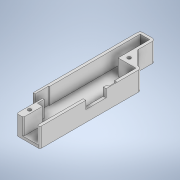
# Autodesk Inventor part: Case_DIP
Saved by Autodesk Inventor 2021 (Build 250183000, 183)
## iProperties
Created: 2021-02-15
Part Number: Case_DIP
Material: Generisch
Document SubType Name: Modeling
Designer: nostrabis
Density: 1 g/cm^3
Appearance: Vorgabe
Author: nostrabis
Autodesk Inventor part; units mm, degrees
ref_plane "YZ Plane" through (0, 0, 0) normal (1, 0, 0) x (0, 1, 0)
ref_plane "XZ Plane" through (0, 0, 0) normal (0, 1, 0) x (-1, 0, 0)
ref_plane "XY Plane" through (0, 0, 0) normal (0, 0, 1) x (1, 0, 0)
sketch "Skizze1" plane through (0, 0, 0) normal (0, 1, 0) x (-1, 0, 0)
  line L0 (0, 0) -> (10, 0)
  line L1 (20, -14) -> (20, -70)
  line L2 (13, -70) -> (0, -70)
  line L3 (0, -70) -> (0, 0)
  line L4 (20, -70) -> (13, -70)
  line L5 (13, -70) -> (13, -93)
  line L6 (13, -93) -> (20, -93)
  line L7 (20, -93) -> (20, -70)
  line L8 (20, 0) -> (10, 0)
  line L9 (10, 0) -> (10, -14)
  line L10 (10, -14) -> (20, -14)
  line L11 (20, -14) -> (20, 0)
  line L12 (20, -12) -> (12, -12)
  line L13 (12, -12) -> (12, 0)
  line L14 (10, 2) -> (-2, 2)
  line L15 (-2, 2) -> (-2, -72)
  line L16 (-2, -72) -> (13, -72)
  line L17 (11, -70) -> (11, -95)
  line L18 (11, -95) -> (22, -95)
  line L19 (22, -95) -> (22, -70)
  line L20 (10, 2) -> (12, 2)
  line L21 (12, 2) -> (12, 0)
  line L22 (20, -12) -> (22, -12)
  line L23 (22, -12) -> (22, -70)
  line L24 (10, 0) -> (10, 2)
  line L25 (0, 0) -> (0, 2)
  line L26 (10, -14) -> (20, -14)
  line L27 (20, -14) -> (20, -21)
  line L28 (20, -21) -> (10, -21)
  line L29 (10, -21) -> (10, -14)
  line L30 (12, -12) -> (12, -14)
  line L31 (20, -21) -> (22, -21)
  line L32 (20, -14) -> (22, -14)
  line L33 (12, 2) -> (15, 2)
  line L34 (15, 2) -> (15, -14)
  line L35 (15, -14) -> (12, -14)
  line L36 (12, -14) -> (12, 2)
  line L37 (10, -14) -> (15, -14)
  line L38 (15, -14) -> (15, -21)
  line L39 (15, -21) -> (10, -21)
  line L40 (10, -21) -> (10, -14)
  point P0 (11, -72)
  dimension "d0" = 20
  dimension "d1" = 70
  dimension "d2" = 7
  dimension "d3" = 23
  dimension "d4" = 10
  dimension "d5" = 14
  dimension "d6" = 2
  dimension "d7" = 2
  dimension "d8" = 2
  dimension "d13" = 7
  constraints: 82 end point, 14 parallel, 10 perpendicular, 8 horizontal, 5 point on line, 2 midpoint, 2 vertical, 1 collinear, 5 other
  measures "d0" distance of L1.end L2.end
  measures "d1" distance of L8.start L1.end
  measures "d2" distance of L6.end L5.end
  measures "d3" distance of L2.start L5.end
  measures "d4" distance of L1.start L9.end
  measures "d5" distance of L0.end L9.end
  measures "d6" distance between parallel lines of L10 L12
  measures "d7" distance between parallel lines of L3 L15
  measures "d8" distance between parallel lines of L5 L17
  measures "d13" distance of L28.end L9.end
extrude "Extrusion1" add sketch "Skizze1" along normal blind 12 contours L3 L2 L17 L16 L15 L14 L25 | L24 L20 L21 L8 | L8 L13 L30 L10 L9 | L21 L33 L34 L8 | L8 L34 L12 L13 | L2 L5 L16 L17 | L12 L34 L10 L30 | L16 L5 L6 L7 L1 L31 L23 L19 L18 L17 | L32 L23 L31 L1
extrude "Extrusion3" add sketch "Skizze1" against normal blind 2 contours L25 L14 L24 L0 | L0 L9 L29 L28 L1 L4 L2 L3 | L3 L2 L17 L16 L15 L14 L25 | L24 L20 L21 L8 | L8 L13 L30 L10 L9 | L21 L33 L34 L8 | L8 L34 L12 L13 | L10 L38 L28 L29 | L2 L5 L16 L17 | L12 L34 L10 L30 | L4 L7 L6 L5 | L16 L5 L6 L7 L1 L31 L23 L19 L18 L17 | L10 L1 L28 L38 | L32 L23 L31 L1
chamfer "Fase1" distance 10 angle 45 1 edges at (-11, 5, -72)
fillet "Rundung1" radius 2 2 edges at (2, 5, -72) (-11, 5, -82)
fillet "Rundung2" radius 2 1 edges at (-1, 5, -72)
fillet "Rundung3" radius 2 2 edges at (-11, 5, -95) (-22, 5, -95)
fillet "Rundung4" radius 1 4 edges at (2, 5, 2) (0, 6, 2) (-10, 6, 2) (-15, 5, 2)
sketch "Skizze4" plane through (0, 12, 0) normal (0, 1, 0) x (1, 0, 0)
  line L0 (-13, 70) -> (0, 70) projected
  line L1 (2, -1) -> (2, 70) projected
  line L2 (0, 70) -> (2, 70)
  line L3 (2, 70) -> (2, 46.2)
  line L4 (2, 46.2) -> (0, 46.2)
  line L5 (0, 46.2) -> (0, 70)
  line L6 (0, 46.2) -> (2, 46.2)
  line L7 (2, 46.2) -> (2, 31.5)
  line L8 (2, 31.5) -> (0, 31.5)
  line L9 (0, 31.5) -> (0, 46.2)
  line L10 (0, 72) -> (-0.1716, 72) projected
  point P0 (0, 0)
  point P1 (2, 31.5)
  dimension "d24" = 14.7
  dimension "d56" = 23.8
  constraints: 16 end point, 4 parallel, 2 horizontal, 2 perpendicular, 2 point on line
  measures "d24" distance of L6.end L7.end
  measures "d56" distance between parallel lines of L0 L4
extrude "Extrusion4" cut sketch "Skizze4" against normal blind 5.8 contours L8 L9 L4 L1
fillet "Rundung5" radius 1 1 edges at (-22, 5, -14)
sketch "Skizze5" plane through (0, -2, 0) normal (0, -1, 0) x (1, 0, 0)
  line L0 (-10, -14) -> (-15, -14) projected
  line L1 (-22, -15) -> (-22, -93) projected
  line L2 (-15, -14) -> (-22, -14)
  line L3 (-22, -14) -> (-22, -17)
  line L4 (-22, -17) -> (-15, -17)
  line L5 (-15, -17) -> (-15, -14)
  point P0 (0, 0)
  dimension "d28" = 3
  constraints: 8 end point, 2 parallel, 1 horizontal, 1 perpendicular, 1 point on line
  measures "d28" distance of L3.end L2.end
extrude "Extrusion5" cut sketch "Skizze5" against normal through all
sketch "Skizze6" plane through (-10, 12, -14) normal (0, 0, -1) x (-1, 0, 0)
  line L0 (0, -12) -> (0, 0) projected
  line L1 (5, -12) -> (5, 0) projected
  line L2 (0, -12) -> (5, -12)
  line L3 (5, -12) -> (5, 0)
  line L4 (5, 0) -> (0, 0)
  line L5 (0, 0) -> (0, -12)
  point P0 (-10, -12)
  constraints: 8 end point, 2 parallel, 1 horizontal, 1 perpendicular
extrude "Extrusion6" add sketch "Skizze6" along normal blind 3
sketch "Skizze7" plane through (0, 12, 0) normal (0, 1, 0) x (1, 0, 0)
  line L0 (-10, -1) -> (-10, 17) projected
  line L1 (-10, 17) -> (-13.8, 17)
  line L2 (-13.8, 17) -> (-13.8, 12)
  line L3 (-13.8, 12) -> (-10, 12)
  line L4 (-10, 12) -> (-10, 17)
  point P0 (0, 0)
  dimension "d34" = 5
  dimension "d35" = 3.8
  constraints: 8 end point, 2 parallel, 1 horizontal, 1 perpendicular
  measures "d34" distance of L1.end L2.end
  measures "d35" distance of L2.end L3.end
extrude "Extrusion7" cut sketch "Skizze7" against normal up to surface (12 mm away)
sketch "Skizze8" plane through (0, 12, 0) normal (0, 1, 0) x (1, 0, 0)
  line L0 (-13, 70) -> (0, 70) projected
  line L1 (-13, 93) -> (-13, 70) projected
  point P0 (0, 0)
  point P1 (-9, 74)
  dimension "d38" = 4
  dimension "d39" = 4
  measures "d38" distance from line of L0 point (-9, 74)
  measures "d39" distance from line of L1 point (-9, 74)
hole "Bohrung1" at (-9, 12, -74) direction (0, -1, 0) diameter 2.5 end through all
sketch "Skizze9" plane through (0, 12, 0) normal (0, 1, 0) x (1, 0, 0)
  line L0 (-10, -1) -> (-10, 12) projected
  line L1 (-14, -2) -> (-11, -2) projected
  point P0 (0, 0)
  point P1 (-12.5, 5)
  dimension "d47" = 2.5
  dimension "d48" = 7
  measures "d47" distance from line of L0 point (-12.5, 5)
  measures "d48" distance from line of L1 point (-12.5, 5)
hole "Bohrung2" at (-12.5, 12, -5) direction (0, -1, 0) diameter 2.5 end through all
sketch "Skizze10" plane through (0, 12, 0) normal (0, 1, 0) x (1, 0, 0)
  line L0 (0, 70) -> (0, 46.2) projected
  line L1 (0, 48.85) -> (1.5, 48.85)
  line L2 (1.5, 48.85) -> (1.5, 54.35)
  line L3 (1.5, 54.35) -> (0, 54.35)
  line L4 (0, 54.35) -> (0, 48.85)
  line L5 (-13, 70) -> (0, 70) projected
  point P0 (0, 0)
  point P1 (0, 54.35)
  dimension "d58" = 5.5
  dimension "d59" = 1.5
  dimension "d60" = 15.65
  constraints: 8 end point, 2 parallel, 1 horizontal, 1 perpendicular, 1 point on line
  measures "d58" distance of L2.end L1.end
  measures "d59" distance between parallel lines of L0 L2
  measures "d60" distance between parallel lines of L5 L3
extrude "Extrusion8" cut sketch "Skizze10" against normal up to surface (12 mm away)
sketch "Skizze11" plane through (0, 12, 0) normal (0, 1, 0) x (1, 0, 0)
  line L0 (-20, 17) -> (-20, 93) projected
  line L1 (-20, 17) -> (-20.5, 17)
  line L2 (-20.5, 17) -> (-20.5, 27)
  line L3 (-20.5, 27) -> (-20, 27)
  line L4 (-20, 27) -> (-20, 17)
  point P0 (0, 0)
  dimension "d63" = 0.5
  dimension "d64" = 10
  constraints: 8 end point, 2 parallel, 1 horizontal, 1 perpendicular
  measures "d63" distance of L2.end L3.end
  measures "d64" distance of L1.end L2.end
extrude "Extrusion9" cut sketch "Skizze11" against normal up to surface (12 mm away)
